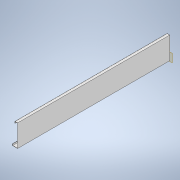
# Autodesk Inventor part: Part2
Saved by Autodesk Inventor 2020 (Build 240168000, 168)
## iProperties
Created: 2022-11-24
Part Number: Part2
Material: Generic
Document SubType Name: Modeling
Designer: super
Density: 1 g/cm^3
Appearance: Default
Author: super
Autodesk Inventor part; units mm, degrees
ref_plane "YZ Plane" through (0, 0, 0) normal (1, 0, 0) x (0, 1, 0)
ref_plane "XZ Plane" through (0, 0, 0) normal (0, 1, 0) x (-1, 0, 0)
ref_plane "XY Plane" through (0, 0, 0) normal (0, 0, 1) x (1, 0, 0)
ref_plane "Work Plane1" through (-50.6614, 0, -158.5) normal (0, 0, 1) x (1, 0, 0)
sketch "Sketch1" plane through (-50.6614, 0, -158.5) normal (0, 0, 1) x (1, 0, 0)
  line L0 (147.1948, -113.8946) -> (147.1948, 236.1054)
  line L1 (147.1948, 236.1054) -> (105.1833, 236.1054)
  line L2 (105.1833, 236.1054) -> (105.1833, 211.1054)
  line L3 (147.1948, -113.8946) -> (67.1948, -113.8946)
  line L4 (67.1948, -113.8946) -> (67.1948, -88.8946)
  line L5 (108.6833, 211.1054) -> (108.6833, 232.6054)
  line L6 (108.6833, 232.6054) -> (143.6948, 232.6054)
  line L7 (143.6948, 232.6054) -> (143.6948, -110.3946)
  line L8 (143.6948, -110.3946) -> (70.6948, -110.3946)
  line L9 (70.6948, -110.3946) -> (70.6948, -88.8946)
  line L10 (67.1948, -88.8946) -> (70.6948, -88.8946)
  line L11 (105.1833, 211.1054) -> (108.6833, 211.1054)
  dimension "d2" = 25
  dimension "d4" = 80
  dimension "d5" = 25
  dimension "d6" = 3.5
  dimension "d7" = 350
  constraints: 24 end point, 6 perpendicular, 2 horizontal, 1 parallel, 1 vertical, 4 other
  measures "d2" distance of L1.end L2.end
  measures "d4" distance of L0.start L3.end
  measures "d5" distance of L3.end L4.end
  measures "d6" distance between parallel lines of L0 L7
  measures "d7" distance of L0.start L0.end
extrude "Extrusion2" add sketch "Sketch1" along normal blind 2400
body "Solid2"
